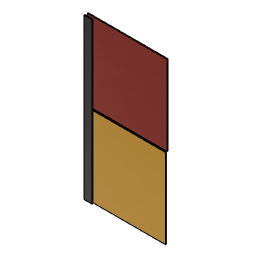
door_attempt (Autodesk Fusion 360 design; units mm, degrees)
Autodesk Fusion 360 part; units mm, degrees
sketch "frame" plane through (0, 0, 0) normal (0, 1, 0) x (1, 0, 0) in component "frame"
  line L0 (0, 0) -> (10, 0)
  line L1 (10, 0) -> (10, -200)
  line L2 (10, -200) -> (0, -200)
  line L3 (0, -200) -> (0, 0)
  dimension "d1" = 10
  dimension "d2" = 200
  constraint horizontal L0
  constraint vertical L1
  constraint horizontal L2
  constraint vertical L3
  constraint coincident L0.start L3.end
  measures "d1" distance of L0.start L0.end
  measures "d2" distance of L0.start L2.end
extrude "Extrude1" add sketch "frame" along normal blind 1 makes body 1 in component "frame"
sketch "frame pins" plane through (0, 1, 0) normal (0, 1, 0) x (-1, 0, 0) in component "frame"
  line L0 (0, 200) -> (-10, 200)
  line L1 (-10, 200) -> (-10, 0)
  line L2 (-10, 0) -> (0, 0)
  line L3 (0, 0) -> (0, 200)
  circle A0 centre (-5, 5) radius 1.25
  line L4 (-10, 0) -> (0, 0)
  line L5 (0, 0) -> (0, 10)
  line L6 (0, 10) -> (-10, 10)
  line L7 (-10, 10) -> (-10, 0)
  line L8 (-10, 200) -> (0, 200)
  line L9 (0, 200) -> (0, 190)
  line L10 (0, 190) -> (-10, 190)
  line L11 (-10, 190) -> (-10, 200)
  line L12 (-10, 200) -> (0, 190)
  circle A1 centre (-5, 195) radius 1.25
  dimension "d5" = 2.5
  dimension "d6" = 2.5
  constraint horizontal L4
  constraint vertical L5
  constraint horizontal L6
  constraint vertical L7
  constraint coincident L3 L5.end
  constraint coincident L1.end L2.start
  constraint horizontal L8
  constraint vertical L9
  constraint horizontal L10
  constraint vertical L11
  constraint coincident L3 L9.end
  constraint coincident L0.end L1.start
  constraint midpoint L12 A1.centre
  measures "d5" diameter of A0
  measures "d6" diameter of A1
extrude "Extrude2" add sketch "frame pins" along normal blind 5 contours L12 A1 | L12 A1 | A0 bodies 1 in component "frame"
sketch "lower door" plane through (0, 0, 0) normal (0, 1, 0) x (1, 0, 0) in component "lower door"
  line L0 (0, 0) -> (100, 0)
  line L1 (100, 0) -> (100, -100)
  line L2 (100, -100) -> (0, -100)
  line L3 (0, -100) -> (0, 0)
  line L4 (10, -10) -> (0, -10)
  line L5 (0, -10) -> (0, 0)
  line L6 (0, 0) -> (10, 0)
  line L7 (10, 0) -> (10, -10)
  line L8 (10, -10) -> (0, 0)
  circle A0 centre (5, -5) radius 1.25
  dimension "d9" = 100
  dimension "d10" = 100
  dimension "d11" = 2.5
  constraint horizontal L0
  constraint vertical L1
  constraint horizontal L2
  constraint vertical L3
  constraint coincident L0.start L3.end
  constraint horizontal L4
  constraint vertical L5
  constraint horizontal L6
  constraint vertical L7
  constraint midpoint L8 A0.centre
  measures "d9" distance of L0.start L0.end
  measures "d10" distance of L0.start L2.end
  measures "d11" diameter of A0
extrude "Extrude1'" add sketch "lower door" along normal blind 3 and the other way blind -2 separate body contours L3 L4 L5 L8 A0 | L0 L6 L7 L8 A0 | L0 L1 L2 L3 L4 L7 makes body 2 in component "lower door"
sketch "upper door" plane through (0, 6, 0) normal (0, 1, 0) x (-1, 0, 0) in component "upper_door"
  circle A0 centre (-5, 5) radius 1.25
  line L0 (-100, 200) -> (0, 200)
  line L1 (0, 200) -> (0, 100)
  line L2 (0, 100) -> (-100, 100)
  line L3 (-100, 100) -> (-100, 200)
  line L4 (0, 200) -> (-10, 200)
  line L5 (-10, 200) -> (-10, 190)
  line L6 (-10, 190) -> (0, 190)
  line L7 (0, 190) -> (0, 200)
  line L8 (-10, 200) -> (0, 190)
  circle A1 centre (-5, 195) radius 1.25
  dimension "d16" = 2.5
  constraint horizontal L0
  constraint vertical L1
  constraint horizontal L2
  constraint vertical L3
  constraint horizontal L4
  constraint vertical L5
  constraint horizontal L6
  constraint vertical L7
  constraint midpoint L8 A1.centre
  measures "d16" diameter of A1
extrude "Extrude1''" add sketch "upper door" along normal blind -2 and the other way blind 1 separate body contours L0 L1 L2 L3 L5 L6 | L5 L6 L8 A1 | L0 L1 L4 L7 L8 A1 makes body 3 in component "upper_door"
sketch "lower door pins" plane through (0, 3, 0) normal (0, 1, 0) x (-1, 0, 0) in component "lower door"
  circle A0 centre (-5, 5) radius 1.25
  line L0 (0, 0) -> (0, 100)
  line L1 (0, 100) -> (-100, 100)
  line L2 (-100, 100) -> (-100, 0)
  line L3 (-100, 0) -> (0, 0)
  line L4 (-100, 0) -> (-60, 0)
  line L5 (-60, 0) -> (-60, 40)
  line L6 (-60, 40) -> (-100, 40)
  line L7 (-100, 40) -> (-100, 0)
  circle A1 centre (-80, 20) radius 2.5
  line L8 (0, 100) -> (-40, 100)
  line L9 (-40, 100) -> (-40, 60)
  line L10 (-40, 60) -> (0, 60)
  line L11 (0, 60) -> (0, 100)
  circle A2 centre (-20, 80) radius 2.5
  dimension "d21" = 40
  dimension "d22" = 40
  dimension "d23" = 5
  dimension "d24" = 40
  dimension "d25" = 40
  dimension "d26" = 5
  constraint horizontal L4
  constraint vertical L5
  constraint horizontal L6
  constraint vertical L7
  constraint coincident L2.end L3.start
  constraint horizontal L8
  constraint vertical L9
  constraint horizontal L10
  constraint vertical L11
  constraint coincident L0.end L1.start
  measures "d21" distance of L2.end L4.end
  measures "d22" distance of L2.end L6.end
  measures "d23" diameter of A1
  measures "d24" distance of L0.end L8.end
  measures "d25" distance of L0.end L10.end
  measures "d26" diameter of A2
extrude "Extrude2'" add sketch "lower door pins" along normal blind 7 contours A1 | A2 bodies 2 in component "lower door"
sketch "upper door pins" plane through (0, 5, 0) normal (0, 1, 0) x (-1, 0, 0) in component "upper_door"
  circle A0 centre (-5, 195) radius 1.25
  line L0 (0, 100) -> (0, 200)
  line L1 (0, 200) -> (-100, 200)
  line L2 (-100, 200) -> (-100, 100)
  line L3 (-100, 100) -> (0, 100)
  line L4 (-100, 200) -> (-60, 200)
  line L5 (-60, 200) -> (-60, 160)
  line L6 (-60, 160) -> (-100, 160)
  line L7 (-100, 160) -> (-100, 200)
  line L8 (0, 100) -> (-40, 100)
  line L9 (-40, 100) -> (-40, 140)
  line L10 (-40, 140) -> (0, 140)
  line L11 (0, 140) -> (0, 100)
  circle A1 centre (-80, 180) radius 2.5
  circle A2 centre (-20, 120) radius 2.5
  dimension "d29" = 40
  dimension "d30" = 40
  dimension "d31" = 40
  dimension "d32" = 40
  dimension "d33" = 5
  dimension "d34" = 5
  constraint horizontal L4
  constraint vertical L5
  constraint horizontal L6
  constraint vertical L7
  constraint coincident L1.end L2.start
  constraint horizontal L8
  constraint vertical L9
  constraint horizontal L10
  constraint vertical L11
  constraint coincident L0.start L3.end
  measures "d29" distance of L1.end L4.end
  measures "d30" distance of L1.end L6.end
  measures "d31" distance of L0.start L8.end
  measures "d32" distance of L0.start L10.end
  measures "d33" diameter of A1
  measures "d34" diameter of A2
extrude "Extrude2''" add sketch "upper door pins" along normal blind 5 contours A1 | A2 bodies 3 in component "upper_door"
sketch "rod" plane through (0, 5, 0) normal (0, 1, 0) x (-1, 0, 0) in component "first_rod"
  circle A0 centre (-80, 180) radius 2.5
  circle A1 centre (-20, 120) radius 2.5
  circle A2 centre (-5, 195) radius 1.25
  line L0 (0, 100) -> (0, 200)
  line L1 (0, 200) -> (-100, 200)
  line L2 (-100, 200) -> (-100, 100)
  line L3 (-100, 100) -> (0, 100)
  line L4 (-100, 200) -> (-60, 200)
  line L5 (-60, 200) -> (-60, 160)
  line L6 (-60, 160) -> (-100, 160)
  line L7 (-100, 160) -> (-100, 200)
  line L8 (0, 100) -> (-40, 100)
  line L9 (-100, 160) -> (-60, 200)
  circle A3 centre (-80, 180) radius 2.5
  line L10 (-40, 100) -> (0, 100)
  line L11 (0, 100) -> (0, 60)
  line L12 (0, 60) -> (-40, 60)
  line L13 (-40, 60) -> (-40, 100)
  line L14 (-40, 100) -> (0, 60)
  circle A4 centre (-20, 80) radius 2.5
  line L15 (-20, 80) -> (-18.2322, 81.7678)
  line L16 (-82.1437, 178.7138) -> (-22.1437, 78.7138)
  line L17 (-77.8563, 181.2862) -> (-17.8563, 81.2862)
  circle A5 centre (-80, 180) radius 3.5
  circle A6 centre (-20, 80) radius 3.5
  line L18 (-80, 180) -> (-32, 100)
  line L19 (-21.8007, 83.0012) -> (-20, 80)
  dimension "d37" = 40
  dimension "d38" = 40
  dimension "d39" = 40
  dimension "d41" = 40
  dimension "d42" = 40
  dimension "d43" = 5
  dimension "d46" = 1
  dimension "d47" = 1
  constraint horizontal L4
  constraint vertical L5
  constraint horizontal L6
  constraint vertical L7
  constraint coincident L1.end L2.start
  constraint horizontal L8
  constraint coincident L0.start L3.end
  constraint concentric A0 A3
  constraint horizontal L10
  constraint vertical L11
  constraint horizontal L12
  constraint vertical L13
  constraint midpoint L14 A4.centre
  constraint coincident A4.centre L15.start
  constraint coincident A4 L15.end
  constraint perpendicular L14 L15
  constraint coincident A0.centre A3.centre
  constraint coincident L3 L18.end
  constraint coincident A6 L19.start
  constraint collinear L18 L19
  measures "d37" distance of L1.end L4.end
  measures "d38" distance of L1.end L6.end
  measures "d39" distance of L0.start L8.end
  measures "d41" distance of L8.end L0.start
  measures "d42" distance of L8.end L12.end
  measures "d43" diameter of A4
extrude "Extrude1'''" add sketch "rod" along normal blind 2 and the other way blind -1 separate body contours A0 A3 L17 A5 L18 | A0 L9 A3 L17 A5 | A0 L9 A3 L16 A5 L18 | A0 L9 A3 L16 A5 | L6 L17 A5 L18 | L6 L16 A5 L18 | L3 L6 L8 L10 L17 L18 | L9 L16 A5 | L3 L6 L8 L10 L16 L18 | L3 L8 L10 L14 L16 L17 A6 | L14 A4 L17 A6 | A4 L17 A6 L19 | L14 A4 A6 L19 | L14 L16 A6 | L14 A4 L16 A6 | L14 A4 L16 A6 makes body 4 in component "first_rod"
move_face "OffsetFaces1" offset -0.3 2 faces at (22.3492, 8.3333, 119.1449) (77.5773, 8.3333, 180.6169) on bodies 3 in component "upper_door"
move_face "OffsetFaces1'" offset -0.3 2 faces at (22.3037, 7.6667, 79.0289) (77.5124, 7.6667, 19.7511) on bodies 2 in component "lower door"
sketch "rod (2)" plane through (0, 5, 0) normal (0, 1, 0) x (-1, 0, 0) in component "second_rod"
  circle A0 centre (-80, 180) radius 2.2
  circle A1 centre (-20, 120) radius 2.2
  circle A2 centre (-5, 195) radius 1.25
  line L0 (0, 100) -> (0, 200)
  line L1 (0, 200) -> (-100, 200)
  line L2 (-100, 200) -> (-100, 100)
  line L3 (-100, 100) -> (0, 100)
  line L4 (0, 100) -> (-40, 100)
  line L5 (-40, 100) -> (-40, 140)
  line L6 (-40, 140) -> (0, 140)
  line L7 (0, 140) -> (0, 100)
  line L8 (-100, 0) -> (-60, 0)
  line L9 (-60, 0) -> (-60, 40)
  line L10 (-60, 40) -> (-100, 40)
  line L11 (-100, 40) -> (-100, 0)
  circle A3 centre (-80, 20) radius 2.5
  circle A4 centre (-20, 120) radius 2.5
  line L12 (-20, 120) -> (-80, 20)
  line L13 (-22.1437, 121.2862) -> (-82.1437, 21.2862)
  line L14 (-17.8563, 118.7138) -> (-77.8563, 18.7138)
  circle A5 centre (-80, 20) radius 3.5
  circle A6 centre (-20, 120) radius 3.5
  dimension "d54" = 40
  dimension "d55" = 40
  dimension "d56" = 40
  dimension "d57" = 40
  dimension "d58" = 5
  dimension "d59" = 5
  dimension "d60" = 2.5
  dimension "d61" = -2.5
  dimension "d62" = 1
  dimension "d63" = 1
  constraint horizontal L4
  constraint vertical L5
  constraint horizontal L6
  constraint vertical L7
  constraint coincident L0.start L3.end
  constraint horizontal L8
  constraint vertical L9
  constraint horizontal L10
  constraint vertical L11
  constraint concentric A1 A4
  constraint coincident A1.centre A4.centre
  constraint coincident A3.centre L12.end
  measures "d54" distance of L0.start L4.end
  measures "d55" distance of L0.start L6.end
  measures "d56" distance of L8.start L8.end
  measures "d57" distance of L8.start L10.end
  measures "d58" diameter of A3
  measures "d59" diameter of A4
extrude "Extrude1''''" add sketch "rod (2)" along normal blind 4 and the other way blind -3 separate body contours L3 L4 L10 L12 L14 | L3 L4 L12 L14 A6 | L3 L4 L10 L12 L13 | L3 L4 L12 L13 A6 | A4 L12 L14 A6 | A4 L13 L14 A6 | L10 L12 L14 A5 | A4 L12 L13 A6 | L10 L12 L13 A5 | A3 L13 L14 A5 | A3 L12 L14 A5 | A3 L12 L13 A5 makes body 5 in component "second_rod"
component "frame" placed x (1, 0, 0) y (0, 1, 0) z (0, 0, 1) at (0, 0, 0)
component "lower door" placed x (1, 0, 0) y (0, 1, 0) z (0, 0, 1) at (0, 0, 0)
component "upper_door" placed x (1, 0, 0) y (0, 1, 0) z (0, 0, 1) at (0, 0, 0)
component "first_rod" placed x (1, 0, 0) y (0, 1, 0) z (0, 0, 1) at (0, 0, 0)
component "second_rod" placed x (1, 0, 0) y (0, 1, 0) z (0, 0, 1) at (0, 0, 0)
named bodies: "frame", "lower door", "upper door", "rod"
